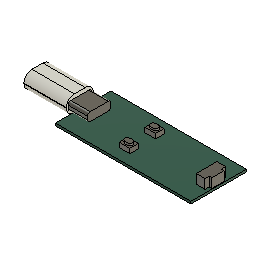
dimmer-control-box-v12 (Autodesk Fusion 360 archive; units mm, degrees)
design "rp2040-plus-board"
Autodesk Fusion 360 part; units mm, degrees
sketch "Sketch1" plane through (0, 0, 0) normal (0, 0, 1) x (1, 0, 0)
  line L0 (-46.4099, -85.064) -> (4.5901, -85.064)
  line L1 (4.5901, -85.064) -> (4.5901, -105.964)
  line L2 (4.5901, -105.964) -> (-46.4099, -105.964)
  line L3 (-46.4099, -105.964) -> (-46.4099, -85.064)
  dimension "d696" = 51
  dimension "d697" = 20.9
  constraint horizontal L0
  constraint vertical L1
  constraint horizontal L2
  constraint vertical L3
  measures "d696" distance of L0.start L0.end
  measures "d697" distance of L0.start L2.end
extrude "Extrude1" add sketch "Sketch1" along normal blind 0.9 makes body 1
sketch "Sketch1 (2)" plane through (-46.4099, 0, 0) normal (-1, 0, 0) x (0, -1, 0) in component "usb-c-port"
  line L0 (85.064, 0) -> (105.964, 0)
  line L1 (105.964, 0) -> (105.964, 0.9)
  line L2 (105.964, 0.9) -> (85.064, 0.9)
  line L3 (85.064, 0.9) -> (85.064, 0)
  line L4 (85.064, 0.9) -> (105.964, 0.9)
  line L5 (95.514, 0.9) -> (95.514, 4.1)
  line L6 (95.514, 2.5) -> (99.914, 2.5)
  line L7 (95.514, 2.5) -> (91.114, 2.5)
  line L8 (91.114, 2.5) -> (91.114, 4.1)
  line L9 (99.914, 2.5) -> (99.914, 0.9)
  line L10 (91.114, 4.1) -> (99.914, 4.1)
  line L11 (99.914, 4.1) -> (99.914, 0.9)
  line L12 (99.914, 0.9) -> (91.114, 0.9)
  line L13 (91.114, 0.9) -> (91.114, 4.1)
  line L14 (99.914, 2.5) -> (99.914, 3)
  line L15 (99.914, 3) -> (99.914, 2)
  line L16 (91.114, 2.5) -> (91.114, 3)
  line L17 (91.114, 3) -> (91.114, 2)
  dimension "d700" = 3.2
  dimension "d701" = 4.4
  dimension "d702" = 4.4
  dimension "d703" = 1.6
  dimension "d704" = 0.5
  dimension "d705" = 1
  dimension "d706" = 0.5
  dimension "d707" = 1
  constraint coincident L2.end L3.start
  constraint coincident L1.end L2.start
  constraint midpoint L4 L5.start
  constraint perpendicular L4 L5
  constraint midpoint L5 L6.start
  constraint perpendicular L5 L6
  constraint parallel L6 L7
  constraint perpendicular L0 L8
  constraint coincident L4 L9.end
  constraint perpendicular L4 L9
  constraint horizontal L10
  constraint vertical L11
  constraint horizontal L12
  constraint vertical L13
  constraint perpendicular L6 L14
  constraint parallel L9 L15
  constraint perpendicular L7 L16
  constraint parallel L13 L17
  measures "d700" distance of L5.start L5.end
  measures "d701" distance of L6.start L6.end
  measures "d702" distance of L6.start L7.end
  measures "d703" distance of L7.end L8.end
  measures "d704" distance of L6.end L14.end
  measures "d705" distance of L14.end L15.end
  measures "d706" distance of L7.end L16.end
  measures "d707" distance of L16.end L17.end
extrude "Extrude1'" add sketch "Sketch1 (2)" against normal blind 7.3 separate body contours L2 L4 L5 L7 L12 L13 L17 | L2 L4 L5 L6 L9 L11 L12 L15 | L5 L7 L8 L10 L13 L16 L17 | L5 L6 L10 L11 L14 L15 makes body 2 in component "usb-c-port"
fillet "Fillet1" radius 1 4 edges at (-42.7599, -91.114, 4.1) (-42.7599, -99.914, 4.1) (-42.7599, -91.114, 0.9) (-42.7599, -99.914, 0.9) on bodies 2 in component "usb-c-port"
sketch "Sketch1 (3)" plane through (-47.6599, 0, 0) normal (-1, 0, 0) x (0, -1, 0) in component "usb-cable-end"
  arc A0 (98.914, 0.9) -> (99.914, 1.9) centre (98.914, 1.9) ccw
  line L0 (99.914, 1.9) -> (99.914, 3.1)
  arc A1 (99.914, 3.1) -> (98.914, 4.1) centre (98.914, 3.1) ccw
  line L1 (98.914, 4.1) -> (92.114, 4.1)
  arc A2 (92.114, 4.1) -> (91.114, 3.1) centre (92.114, 3.1) ccw
  line L2 (91.114, 3.1) -> (91.114, 1.9)
  arc A3 (91.114, 1.9) -> (92.114, 0.9) centre (92.114, 1.9) ccw
  line L3 (92.114, 0.9) -> (98.914, 0.9)
  line L4 (95.514, 4.1) -> (95.514, 0.9)
  line L5 (91.114, 2.5) -> (99.914, 2.5)
  line L6 (95.514, 2.5) -> (95.514, 5.6)
  line L7 (95.514, 2.5) -> (95.514, -0.6)
  line L8 (95.514, 2.5) -> (100.564, 2.5)
  line L9 (95.514, 2.5) -> (90.464, 2.5)
  line L10 (90.464, 2.5) -> (90.464, 5.6)
  line L11 (100.564, 2.5) -> (100.564, -0.6)
  line L12 (100.564, -0.6) -> (90.464, -0.6)
  line L13 (90.464, -0.6) -> (90.464, 5.6)
  line L14 (90.464, 5.6) -> (100.564, 5.6)
  line L15 (100.564, 5.6) -> (100.564, -0.6)
  dimension "d725" = 3.1
  dimension "d726" = 3.1
  dimension "d727" = 5.05
  dimension "d728" = 5.05
  dimension "d729" = 3.1
  dimension "d730" = 3.1
  constraint midpoint L1 L4.start
  constraint midpoint L3 L4.end
  constraint midpoint L2 L5.start
  constraint midpoint L0 L5.end
  constraint midpoint L4 L6.start
  constraint perpendicular L5 L6
  constraint perpendicular L5 L7
  constraint perpendicular L7 L8
  constraint perpendicular L7 L9
  constraint perpendicular L9 L10
  constraint perpendicular L8 L11
  constraint horizontal L12
  constraint vertical L13
  constraint horizontal L14
  constraint vertical L15
  measures "d725" distance of L6.start L6.end
  measures "d726" distance of L6.start L7.end
  measures "d727" distance of L6.start L8.end
  measures "d728" distance of L6.start L9.end
  measures "d729" distance of L9.end L10.end
  measures "d730" distance of L8.end L11.end
extrude "Extrude1''" add sketch "Sketch1 (3)" along normal blind 16 separate body makes body 3 in component "usb-cable-end"
fillet "Fillet1'" radius 3 4 edges at (-55.6599, -100.564, 5.6) (-55.6599, -90.464, 5.6) (-55.6599, -90.464, -0.6) (-55.6599, -100.564, -0.6) on bodies 3 in component "usb-cable-end"
sketch "Sketch1 (4)" plane through (0, 0, 0.9) normal (0, 0, 1) x (-1, 0, 0) in component "buttons"
  line L0 (46.4099, 105.964) -> (-4.5901, 105.964)
  line L1 (-4.5901, 105.964) -> (-4.5901, 85.064)
  line L2 (-4.5901, 85.064) -> (46.4099, 85.064)
  line L3 (46.4099, 85.064) -> (46.4099, 105.964)
  line L4 (46.4099, 85.064) -> (26.4099, 85.064)
  line L5 (26.4099, 85.064) -> (26.4099, 105.964)
  line L6 (26.4099, 85.064) -> (26.4099, 89.064)
  line L7 (26.4099, 105.964) -> (26.4099, 101.964)
  line L8 (26.4099, 89.064) -> (22.4099, 89.064)
  line L9 (22.4099, 89.064) -> (22.4099, 92.264)
  line L10 (22.4099, 92.264) -> (26.4099, 92.264)
  line L11 (26.4099, 92.264) -> (26.4099, 89.064)
  line L12 (26.4099, 101.964) -> (22.4099, 101.964)
  line L13 (22.4099, 101.964) -> (22.4099, 98.764)
  line L14 (22.4099, 98.764) -> (26.4099, 98.764)
  line L15 (26.4099, 98.764) -> (26.4099, 101.964)
  line L16 (26.4099, 90.664) -> (24.4099, 90.664)
  line L17 (26.4099, 100.364) -> (24.4099, 100.364)
  line L18 (24.4099, 100.364) -> (24.4099, 99.314)
  line L19 (24.4099, 90.664) -> (24.4099, 89.614)
  line L20 (24.4099, 90.664) -> (22.9099, 90.664)
  line L21 (24.4099, 100.364) -> (22.9099, 100.364)
  ellipse E0 centre (24.4099, 100.364) end of major axis (22.9099, 100.364) minor radius 1.05
  line L22 (25.9099, 100.364) -> (22.9099, 100.364) construction
  line L23 (24.4099, 101.414) -> (24.4099, 99.314) construction
  ellipse E1 centre (24.4099, 90.664) end of major axis (22.9099, 90.664) minor radius 1.05
  line L24 (25.9099, 90.664) -> (22.9099, 90.664) construction
  line L25 (24.4099, 91.714) -> (24.4099, 89.614) construction
  dimension "d432" = 20
  dimension "d433" = 4
  dimension "d434" = 4
  dimension "d435" = 4
  dimension "d436" = 3.2
  dimension "d437" = 4
  dimension "d438" = 3.2
  dimension "d439" = 2
  dimension "d440" = 2
  dimension "d441" = 1.05
  dimension "d442" = 1.05
  dimension "d443" = 1.5
  dimension "d444" = 1.5
  constraint coincident L2.end L3.start
  constraint perpendicular L3 L4
  constraint coincident L0 L5.end
  constraint perpendicular L0 L5
  constraint perpendicular L2 L6
  constraint perpendicular L0 L7
  constraint horizontal L8
  constraint vertical L9
  constraint horizontal L10
  constraint vertical L11
  constraint horizontal L12
  constraint vertical L13
  constraint horizontal L14
  constraint vertical L15
  constraint midpoint L11 L16.start
  constraint perpendicular L9 L16
  constraint midpoint L15 L17.start
  constraint perpendicular L5 L17
  constraint perpendicular L17 L18
  constraint perpendicular L16 L19
  constraint perpendicular L19 L20
  constraint perpendicular L18 L21
  constraint coincident E0 L22.start
  constraint coincident L21.end E0
  constraint coincident E0 L23.start
  constraint coincident L18.end E0
  constraint perpendicular L18 L22
  constraint coincident E1 L24.start
  constraint coincident L20.end E1
  constraint coincident E1 L25.start
  constraint coincident L19.end E1
  constraint perpendicular L19 L24
  measures "d432" distance of L2.end L4.end
  measures "d433" distance of L4.end L6.end
  measures "d434" distance of L5.end L7.end
  measures "d435" distance of L6.end L8.end
  measures "d436" distance of L6.end L10.end
  measures "d437" distance of L7.end L12.end
  measures "d438" distance of L7.end L14.end
  measures "d439" distance of L16.start L16.end
  measures "d440" distance of L17.start L17.end
  measures "d441" distance of L17.end L18.end
  measures "d442" distance of L16.end L19.end
  measures "d443" distance of L16.end L20.end
  measures "d444" distance of L17.end L21.end
extrude "Extrude1'''" add sketch "Sketch1 (4)" along normal blind 2.5 separate body contours L16 L19 E1 | L16 L20 E1 | L19 L20 E1 | L17 L18 E0 | L17 L21 E0 | L18 L21 E0 makes body 4 at (-24.3629, -91.7135, 2.5667) makes body 5 at (-24.3629, -101.4135, 2.5667) in component "buttons"
extrude "Extrude2" add sketch "Sketch1 (4)" along normal blind 1.75 contours L5 L12 L13 L14 L15 | L5 L8 L9 L10 L11 bodies 4 5 in component "buttons"
sketch "Sketch1 (5)" plane through (0, 0, 0.9) normal (0, 0, 1) x (-1, 0, 0) in component "connector"
  line L0 (46.4099, 105.964) -> (-4.5901, 105.964)
  line L1 (-4.5901, 105.964) -> (-4.5901, 85.064)
  line L2 (-4.5901, 85.064) -> (46.4099, 85.064)
  line L3 (46.4099, 85.064) -> (46.4099, 105.964)
  line L4 (-4.5901, 95.514) -> (-1.6901, 95.514) construction
  line L5 (-0.0401, 99.414) -> (-3.3401, 99.414)
  line L6 (-3.3401, 99.414) -> (-3.3401, 91.614)
  line L7 (-3.3401, 91.614) -> (-0.0401, 91.614)
  line L8 (-0.0401, 91.614) -> (-0.0401, 99.414)
  line L9 (-0.0401, 99.414) -> (-3.3401, 91.614) construction
  line L10 (-3.3401, 99.414) -> (-0.0401, 91.614) construction
  line L11 (-4.5901, 93.214) -> (-3.3401, 93.214)
  line L12 (-4.5901, 97.814) -> (-3.3401, 97.814)
  line L13 (-4.3401, 97.814) -> (-4.3401, 93.214)
  point P0 (-1.6901, 95.514)
  dimension "d1" = 2.9
  dimension "d2" = 3.3
  dimension "d3" = 7.8
  dimension "d4" = 2.3
  dimension "d5" = -2.3
  dimension "d6" = -0.25
  constraint midpoint L1 L4.start
  constraint perpendicular L1 L4
  constraint horizontal L5
  constraint perpendicular L5 L6
  constraint parallel L5 L7
  constraint parallel L6 L8
  constraint coincident L9 P0
  constraint coincident L10 P0
  constraint coincident P0 L4.end
  constraint coincident L1 L12.start
  constraint coincident L1 L11.start
  constraint coincident L6 L11.end
  constraint coincident L6 L12.end
  constraint coincident L11 L13.end
  constraint coincident L12 L13.start
  measures "d1" distance of L4.start P0
  measures "d2" distance of L6.end L7.end
  measures "d3" distance of L5.end L6.end
extrude "Extrude1''''" add sketch "Sketch1 (5)" along normal blind 3.5 separate body contours L6 L11 L12 L13 | L5 L6 L7 L8 makes body 6 in component "connector"
component "usb-c-port" placed x (1, 0, 0) y (0, 1, 0) z (0, 0, 1) at (-1.25, 0, 0)
component "usb-cable-end" placed x (1, 0, 0) y (0, 1, 0) z (0, 0, 1) at (0, 0, 0)
component "buttons" placed x (1, 0, 0) y (0, 1, 0) z (0, 0, 1) at (0, 0, 0)
component "connector" placed x (1, 0, 0) y (0, 1, 0) z (0, 0, 1) at (0, 0, 0)
equation "d1 = ( ( 3.3 / 2 ) * 1 mm ) + 1.25 mm"
equation "d4 = ( 4.6 / 2 ) * 1 mm"

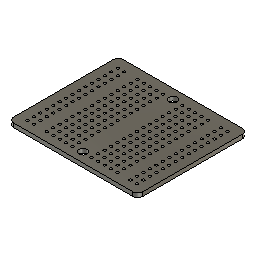
design "dikavs-proto-pcb"
Autodesk Fusion 360 part; units mm, degrees
sketch "Sketch1" plane through (0, 0, 0) normal (0, 0, 1) x (1, 0, 0) in component "pcb"
  line L0 (25.4, -21.55) -> (-25.4, -21.55)
  line L1 (-25.4, -21.55) -> (-25.4, 21.55)
  line L2 (-25.4, 21.55) -> (25.4, 21.55)
  line L3 (25.4, 21.55) -> (25.4, -21.55)
  line L4 (25.4, -21.55) -> (-25.4, 21.55) construction
  line L5 (-25.4, -21.55) -> (25.4, 21.55) construction
  line L6 (0, 17.75) -> (0, -17.75) construction
  circle A0 centre (0, 17.75) radius 1.6
  circle A1 centre (0, -17.75) radius 1.6
  dimension "d1" = 50.8
  dimension "d2" = 43.1
  dimension "d3" = 3.2
  dimension "d4" = 3.2
  dimension "d5" = 35.5
  constraint horizontal L0
  constraint perpendicular L0 L1
  constraint parallel L0 L2
  constraint parallel L1 L3
  constraint coincident L4 origin
  constraint coincident L5 origin
  constraint perpendicular L0 L6
  constraint midpoint origin L6
  constraint coincident L6.start A0.centre
  constraint coincident L6.end A1.centre
  measures "d1" distance of L1.end L2.end
  measures "d2" distance of L0.end L1.end
  measures "d3" diameter of A0
  measures "d4" diameter of A1
  measures "d5" distance of L6.start L6.end
extrude "Extrude1" add sketch "Sketch1" along normal blind 1.6 in component "pcb"
fillet "Fillet1" radius 2 4 edges at (-25.4, -21.55, 0.8) (-25.4, 21.55, 0.8) (25.4, 21.55, 0.8) (25.4, -21.55, 0.8) in component "pcb"
sketch "Sketch2" plane through (0, 0, 1.6) normal (0, 0, 1) x (-1, 0, 0) in component "pcb"
  arc A0 (-23.4, 21.55) -> (-25.4, 19.55) centre (-23.4, 19.55) ccw
  line L0 (-25.4, 19.55) -> (-25.4, -19.55)
  arc A1 (-25.4, -19.55) -> (-23.4, -21.55) centre (-23.4, -19.55) ccw
  line L1 (-23.4, -21.55) -> (23.4, -21.55)
  arc A2 (23.4, -21.55) -> (25.4, -19.55) centre (23.4, -19.55) ccw
  line L2 (25.4, -19.55) -> (25.4, 19.55)
  arc A3 (25.4, 19.55) -> (23.4, 21.55) centre (23.4, 19.55) ccw
  line L3 (23.4, 21.55) -> (-23.4, 21.55)
  circle A4 centre (0, 17.75) radius 1.6
  circle A5 centre (0, -17.75) radius 1.6
  line L4 (0, -21.55) -> (0, 21.55) construction
  line L5 (-3.75, -21.55) -> (-3.75, 21.55) construction
  circle A6 centre (-3.75, -17.55) radius 0.5
  dimension "d10" = -3.75
  dimension "d11" = 1
  dimension "d12" = 4
  constraint midpoint L1 L4.start
  constraint midpoint L3 L4.end
  constraint coincident L1 L5.start
  constraint coincident L3 L5.end
  constraint coincident L5 A6.centre
  measures "d11" diameter of A6
  measures "d12" distance of L1 A6.centre
extrude "Extrude2" cut sketch "Sketch2" against normal blind 1.6 contours A6 in component "pcb"
pattern_linear "R-Pattern1" count 15 spacing 2.54 along (0, -1, 0) count 5 spacing 2.54 along (1, 0, 0) of "Extrude2" in component "pcb"
mirror "Mirror1" about plane through (0, 0, 0) normal (1, 0, 0) of "Extrude2", "R-Pattern1" in component "pcb"
sketch "Sketch3" plane through (0, 0, 1.6) normal (0, 0, 1) x (-1, 0, 0) in component "pcb"
  circle A0 centre (3.75, 7.85) radius 0.5
  circle A1 centre (3.75, 5.31) radius 0.5
  circle A2 centre (6.29, -17.55) radius 0.5
  circle A3 centre (3.75, 15.47) radius 0.5
  circle A4 centre (3.75, 2.77) radius 0.5
  circle A5 centre (3.75, 10.39) radius 0.5
  circle A6 centre (8.83, -2.31) radius 0.5
  circle A7 centre (8.83, 0.23) radius 0.5
  circle A8 centre (8.83, 2.77) radius 0.5
  circle A9 centre (8.83, 5.31) radius 0.5
  circle A10 centre (8.83, 7.85) radius 0.5
  circle A11 centre (8.83, 10.39) radius 0.5
  circle A12 centre (8.83, 12.93) radius 0.5
  circle A13 centre (8.83, 15.47) radius 0.5
  circle A14 centre (8.83, 18.01) radius 0.5
  circle A15 centre (11.37, -17.55) radius 0.5
  circle A16 centre (11.37, -15.01) radius 0.5
  circle A17 centre (11.37, -12.47) radius 0.5
  circle A18 centre (11.37, -9.93) radius 0.5
  circle A19 centre (11.37, -7.39) radius 0.5
  circle A20 centre (11.37, -4.85) radius 0.5
  circle A21 centre (11.37, -2.31) radius 0.5
  circle A22 centre (11.37, 0.23) radius 0.5
  circle A23 centre (11.37, 2.77) radius 0.5
  circle A24 centre (11.37, 5.31) radius 0.5
  circle A25 centre (11.37, 7.85) radius 0.5
  circle A26 centre (11.37, 10.39) radius 0.5
  circle A27 centre (11.37, 12.93) radius 0.5
  circle A28 centre (11.37, 15.47) radius 0.5
  circle A29 centre (11.37, 18.01) radius 0.5
  circle A30 centre (13.91, -17.55) radius 0.5
  circle A31 centre (13.91, -15.01) radius 0.5
  circle A32 centre (13.91, -12.47) radius 0.5
  circle A33 centre (13.91, -9.93) radius 0.5
  circle A34 centre (13.91, -4.85) radius 0.5
  circle A35 centre (13.91, -2.31) radius 0.5
  circle A36 centre (13.91, 0.23) radius 0.5
  circle A37 centre (13.91, 2.77) radius 0.5
  circle A38 centre (13.91, 5.31) radius 0.5
  circle A39 centre (13.91, 7.85) radius 0.5
  circle A40 centre (13.91, 10.39) radius 0.5
  circle A41 centre (13.91, 12.93) radius 0.5
  circle A42 centre (6.29, -12.47) radius 0.5
  circle A43 centre (6.29, -9.93) radius 0.5
  circle A44 centre (6.29, -7.39) radius 0.5
  circle A45 centre (6.29, -4.85) radius 0.5
  circle A46 centre (6.29, -2.31) radius 0.5
  circle A47 centre (6.29, 0.23) radius 0.5
  circle A48 centre (6.29, 2.77) radius 0.5
  circle A49 centre (6.29, 5.31) radius 0.5
  circle A50 centre (6.29, 7.85) radius 0.5
  circle A51 centre (6.29, 10.39) radius 0.5
  circle A52 centre (6.29, 12.93) radius 0.5
  circle A53 centre (6.29, 15.47) radius 0.5
  circle A54 centre (6.29, 18.01) radius 0.5
  circle A55 centre (8.83, -17.55) radius 0.5
  circle A56 centre (8.83, -15.01) radius 0.5
  circle A57 centre (8.83, -12.47) radius 0.5
  circle A58 centre (8.83, -9.93) radius 0.5
  circle A59 centre (8.83, -7.39) radius 0.5
  circle A60 centre (8.83, -4.85) radius 0.5
  circle A61 centre (3.75, 12.93) radius 0.5
  circle A62 centre (3.75, -7.39) radius 0.5
  circle A63 centre (3.75, -4.85) radius 0.5
  circle A64 centre (3.75, 0.23) radius 0.5
  circle A65 centre (3.75, -2.31) radius 0.5
  circle A66 centre (3.75, -15.01) radius 0.5
  circle A67 centre (3.75, -12.47) radius 0.5
  circle A68 centre (3.75, -9.93) radius 0.5
  circle A69 centre (13.91, 15.47) radius 0.5
  circle A70 centre (3.75, 18.01) radius 0.5
  circle A71 centre (13.91, 18.01) radius 0.5
  circle A72 centre (6.29, -15.01) radius 0.5
  circle A73 centre (13.91, -7.39) radius 0.5
  circle A74 centre (3.75, -17.55) radius 0.5
  circle A75 centre (-13.91, 18.01) radius 0.5
  circle A76 centre (-13.91, 15.47) radius 0.5
  circle A77 centre (-13.91, 12.93) radius 0.5
  circle A78 centre (-13.91, 10.39) radius 0.5
  circle A79 centre (-13.91, 7.85) radius 0.5
  circle A80 centre (-13.91, 5.31) radius 0.5
  circle A81 centre (-13.91, 2.77) radius 0.5
  circle A82 centre (-13.91, 0.23) radius 0.5
  circle A83 centre (-13.91, -2.31) radius 0.5
  circle A84 centre (-13.91, -4.85) radius 0.5
  circle A85 centre (-13.91, -7.39) radius 0.5
  circle A86 centre (-13.91, -9.93) radius 0.5
  circle A87 centre (-13.91, -12.47) radius 0.5
  circle A88 centre (-13.91, -15.01) radius 0.5
  circle A89 centre (-13.91, -17.55) radius 0.5
  circle A90 centre (-11.37, 18.01) radius 0.5
  circle A91 centre (-11.37, 15.47) radius 0.5
  circle A92 centre (-11.37, 12.93) radius 0.5
  circle A93 centre (-11.37, 10.39) radius 0.5
  circle A94 centre (-11.37, 7.85) radius 0.5
  circle A95 centre (-11.37, 5.31) radius 0.5
  circle A96 centre (-11.37, 2.77) radius 0.5
  circle A97 centre (-11.37, 0.23) radius 0.5
  circle A98 centre (-11.37, -2.31) radius 0.5
  circle A99 centre (-11.37, -4.85) radius 0.5
  circle A100 centre (-11.37, -7.39) radius 0.5
  circle A101 centre (-11.37, -9.93) radius 0.5
  circle A102 centre (-11.37, -12.47) radius 0.5
  circle A103 centre (-11.37, -15.01) radius 0.5
  circle A104 centre (-11.37, -17.55) radius 0.5
  circle A105 centre (-8.83, 18.01) radius 0.5
  circle A106 centre (-8.83, 15.47) radius 0.5
  circle A107 centre (-8.83, 12.93) radius 0.5
  circle A108 centre (-8.83, 10.39) radius 0.5
  circle A109 centre (-8.83, 7.85) radius 0.5
  circle A110 centre (-8.83, 5.31) radius 0.5
  circle A111 centre (-8.83, 2.77) radius 0.5
  circle A112 centre (-8.83, 0.23) radius 0.5
  circle A113 centre (-8.83, -2.31) radius 0.5
  circle A114 centre (-8.83, -4.85) radius 0.5
  circle A115 centre (-8.83, -7.39) radius 0.5
  circle A116 centre (-8.83, -9.93) radius 0.5
  circle A117 centre (-8.83, -12.47) radius 0.5
  circle A118 centre (-8.83, -15.01) radius 0.5
  circle A119 centre (-8.83, -17.55) radius 0.5
  circle A120 centre (-6.29, 18.01) radius 0.5
  circle A121 centre (-6.29, 15.47) radius 0.5
  circle A122 centre (-6.29, 12.93) radius 0.5
  circle A123 centre (-6.29, 10.39) radius 0.5
  circle A124 centre (-6.29, 7.85) radius 0.5
  circle A125 centre (-6.29, 5.31) radius 0.5
  circle A126 centre (-6.29, 2.77) radius 0.5
  circle A127 centre (-6.29, 0.23) radius 0.5
  circle A128 centre (-6.29, -2.31) radius 0.5
  circle A129 centre (-6.29, -4.85) radius 0.5
  circle A130 centre (-6.29, -7.39) radius 0.5
  circle A131 centre (-6.29, -9.93) radius 0.5
  circle A132 centre (-6.29, -12.47) radius 0.5
  circle A133 centre (-6.29, -15.01) radius 0.5
  circle A134 centre (-6.29, -17.55) radius 0.5
  circle A135 centre (-3.75, 18.01) radius 0.5
  circle A136 centre (-3.75, 15.47) radius 0.5
  circle A137 centre (-3.75, 12.93) radius 0.5
  circle A138 centre (-3.75, 10.39) radius 0.5
  circle A139 centre (-3.75, 7.85) radius 0.5
  circle A140 centre (-3.75, 5.31) radius 0.5
  circle A141 centre (-3.75, 2.77) radius 0.5
  circle A142 centre (-3.75, 0.23) radius 0.5
  circle A143 centre (-3.75, -2.31) radius 0.5
  circle A144 centre (-3.75, -4.85) radius 0.5
  circle A145 centre (-3.75, -7.39) radius 0.5
  circle A146 centre (-3.75, -9.93) radius 0.5
  circle A147 centre (-3.75, -12.47) radius 0.5
  circle A148 centre (-3.75, -15.01) radius 0.5
  circle A149 centre (-3.75, -17.55) radius 0.5
  arc A150 (-23.4, 21.55) -> (-25.4, 19.55) centre (-23.4, 19.55) ccw
  line L0 (-25.4, 19.55) -> (-25.4, -19.55)
  arc A151 (-25.4, -19.55) -> (-23.4, -21.55) centre (-23.4, -19.55) ccw
  line L1 (-23.4, -21.55) -> (23.4, -21.55)
  arc A152 (23.4, -21.55) -> (25.4, -19.55) centre (23.4, -19.55) ccw
  line L2 (25.4, -19.55) -> (25.4, 19.55)
  arc A153 (25.4, 19.55) -> (23.4, 21.55) centre (23.4, 19.55) ccw
  line L3 (23.4, 21.55) -> (-23.4, 21.55)
  circle A154 centre (0, 17.75) radius 1.6
  circle A155 centre (0, -17.75) radius 1.6
  line L4 (-23.4, -21.55) -> (23.4, -21.55)
  line L5 (23.4, 21.55) -> (-23.4, 21.55)
  line L6 (0, 21.55) -> (0, -21.55) construction
  line L7 (-19, 21.55) -> (-19, -21.55) construction
  circle A156 centre (-19, -17.55) radius 0.5
  dimension "d21" = 19
  dimension "d22" = 1
  dimension "d23" = 4
  constraint midpoint L5 L6.start
  constraint midpoint L4 L6.end
  constraint coincident L4 L7.end
  constraint coincident L3 L7.start
  constraint coincident L7 A156.centre
  measures "d22" diameter of A156
  measures "d23" distance of L4 A156.centre
extrude "Extrude3" cut sketch "Sketch3" against normal blind 1.6 contours A156 in component "pcb"
pattern_linear "R-Pattern2" count 15 spacing 2.54 along (0, -1, 0) count 2 spacing 2.54 along (1, 0, 0) of "Extrude3" in component "pcb"
mirror "Mirror2" about plane through (0, 0, 0) normal (1, 0, 0) of "Extrude3", "R-Pattern2" in component "pcb"
component "pcb" placed x (1, 0, 0) y (0, 1, 0) z (0, 0, 1) at (0, 0, 0)
equation "d5 = 32.3 mm + 3.2 mm"

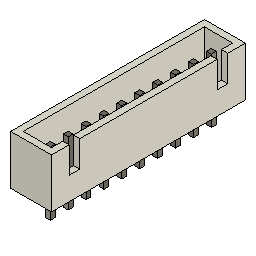
design "JST-XH-socket-10p"
Autodesk Fusion 360 part; units mm, degrees
sketch "Sketch1" plane through (0, 0, 0) normal (0, 0, 1) x (1, 0, 0) in component "socket-body"
  line L0 (2.9, 13.75) -> (-2.9, 13.75)
  line L1 (-2.9, 13.75) -> (-2.9, -13.75)
  line L2 (-2.9, -13.75) -> (2.9, -13.75)
  line L3 (2.9, -13.75) -> (2.9, 13.75)
  line L4 (2.9, 13.75) -> (-2.9, -13.75) construction
  line L5 (-2.9, 13.75) -> (2.9, -13.75) construction
  line L6 (2, -12.85) -> (2, 12.85)
  line L7 (2, 12.85) -> (-2, 12.85)
  line L8 (-2, 12.85) -> (-2, -12.85)
  line L9 (-2, -12.85) -> (2, -12.85)
  dimension "d1" = 5.8
  dimension "d2" = 27.5
  dimension "d3" = -0.9
  constraint horizontal L0
  constraint perpendicular L0 L1
  constraint parallel L0 L2
  constraint parallel L1 L3
  constraint coincident L4 origin
  constraint coincident L5 origin
  measures "d1" distance of L1.end L2.end
  measures "d2" distance of L0.end L1.end
extrude "Extrude1" add sketch "Sketch1" along normal blind 7 makes body 1 in component "socket-body"
extrude "Extrude2" add sketch "Sketch1" along normal blind 0.5 contours L6 L7 L8 L9 bodies 1 in component "socket-body"
sketch "Sketch1 (2)" plane through (0, 0, 0.5) normal (0, 0, 1) x (-1, 0, 0) in component "pins"
  line L0 (2, 12.85) -> (-2, 12.85)
  line L1 (-2, 12.85) -> (-2, -12.85)
  line L2 (-2, -12.85) -> (2, -12.85)
  line L3 (2, -12.85) -> (2, 12.85)
  line L4 (-0.5, 12.85) -> (-0.5, -12.85) construction
  line L5 (-0.85, -1.5174) -> (-0.15, -1.5174)
  line L6 (-0.15, -1.5174) -> (-0.15, -0.8174)
  line L7 (-0.15, -0.8174) -> (-0.85, -0.8174)
  line L8 (-0.85, -0.8174) -> (-0.85, -1.5174)
  line L9 (-0.85, -1.5174) -> (-0.15, -0.8174) construction
  line L10 (-0.15, -1.5174) -> (-0.85, -0.8174) construction
  point P0 (-0.5, -1.1674)
  dimension "d8" = 0.7
  dimension "d9" = 0.7
  dimension "d10" = 1.27
  dimension "d19" = 1.5
  constraint horizontal L5
  constraint perpendicular L5 L6
  constraint parallel L5 L7
  constraint parallel L6 L8
  constraint coincident L9 P0
  constraint coincident L10 P0
  constraint coincident L4 P0
  constraint vertical L4
  constraint coincident L2 L4.end
  constraint coincident L0 L4.start
  measures "d8" distance of L6.end L7.end
  measures "d9" distance of L5.end L6.end
  measures "d10" distance of origin P0
  measures "d19" distance of L1 L4
extrude "Extrude1'" add sketch "Sketch1 (2)" along normal blind 5.5 separate body contours L5 L6 L7 L8 makes body 2 in component "pins"
extrude "Extrude2'" add 1 faces at (0.3833, 1.2841, 0.5) along direction (0, 0, -1) blind 3.5 on bodies 2 bodies 2 in component "pins"
pattern_linear "R-Pattern1" count 10 spacing 2.54 along (0, -1, 0) both ways of "Extrude1'", "Extrude2'" makes body 3 at (0.3833, 10.9774, 0) makes body 4 at (0.85, 8.6708, 0) makes body 5 at (0.3833, 5.8974, 0) makes body 6 at (0.85, 3.5908, 0) makes body 7 at (0.85, -1.4892, 0) makes body 8 at (0.85, -4.0292, 0) makes body 9 at (0.15, -6.5692, 3) makes body 10 at (0.3833, -9.3426, 0) makes body 11 at (0.3833, -11.8826, 0) in component "pins"
sketch "Sketch2" plane through (2.9, 0, 0) normal (1, 0, 0) x (0, 1, 0) in component "socket-body"
  line L0 (-13.75, 0) -> (13.75, 0)
  line L1 (13.75, 0) -> (13.75, 7)
  line L2 (13.75, 7) -> (-13.75, 7)
  line L3 (-13.75, 7) -> (-13.75, 0)
  line L4 (0, 7) -> (0, 0) construction
  line L5 (-13.75, 3.25) -> (-11.25, 3.25) construction
  line L6 (-11.25, 3.25) -> (-9.75, 3.25)
  line L7 (-11.25, 3.25) -> (-11.25, 7)
  line L8 (-9.75, 3.25) -> (-9.75, 7)
  line L9 (11.25, 3.25) -> (11.25, 7)
  line L10 (11.25, 3.25) -> (9.75, 3.25)
  line L11 (9.75, 3.25) -> (9.75, 7)
  dimension "d20" = 2.5
  dimension "d21" = 3.25
  dimension "d22" = 1.5
  constraint midpoint L2 L4.start
  constraint coincident L4.end origin
  constraint coincident L3 L5.start
  constraint perpendicular L3 L5
  constraint parallel L5 L6
  constraint coincident L2 L7.end
  constraint perpendicular L2 L7
  constraint coincident L2 L8.end
  constraint perpendicular L2 L8
  constraint symmetric L4 L5.end L9.start
  constraint symmetric L4 L6.end L10.end
  constraint symmetric L4 L7.end L9.end
  constraint symmetric L4 L8.end L11.end
  measures "d20" distance of L5.start L5.end
  measures "d21" distance of L0.start L5.start
  measures "d22" distance of L5.end L6.end
extrude "Extrude3" cut sketch "Sketch2" against normal blind 1 contours L2 L6 L7 L8 | L2 L9 L10 L11 bodies 1 in component "socket-body"
component "socket-body" placed x (1, 0, 0) y (0, 1, 0) z (0, 0, 1) at (0, 0, 0)
component "pins" placed x (1, 0, 0) y (0, 1, 0) z (0, 0, 1) at (0, 0, 0) in component "socket-body"
equation "d10 = ( 2.54 / 2 ) * 1 mm"
